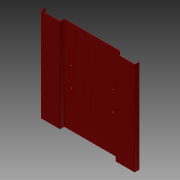
# Autodesk Inventor part: foot
Saved by Autodesk Inventor 2014 SP2 (Build 180246200, 246)
## iProperties
Created: 2016-09-27
Part Number: foot
Material: Steel, Mild
Document SubType Name: Sheet Metal
Designer: cruiser
Density: 7.86 g/cm^3
Sheet Metal Rule: Default_mm
Appearance: Red
Mass: 553.617 g
Surface Area: 901.353 cm^2
Volume: 70.4348 cm^3
Flat Pattern Width: 19.6 cm
Flat Pattern Length: 23.0315 cm
Flat Pattern Area: 451.417 cm^2
Sheet Metal Width: 196.000 mm
Sheet Metal Length: 230.315 mm
Sheet Metal Area: 45141.652 mm^2
Author: cruiser
Autodesk Inventor part; units mm, degrees
ref_plane "YZ Plane" through (0, 0, 0) normal (1, 0, 0) x (0, 1, 0)
ref_plane "XZ Plane" through (0, 0, 0) normal (0, 1, 0) x (-1, 0, 0)
ref_plane "XY Plane" through (0, 0, 0) normal (0, 0, 1) x (1, 0, 0)
sketch "Sketch1" plane through (0, 0, 0) normal (0, 1, 0) x (-1, 0, 0)
  line L0 (-59, -98) -> (59, -98)
  line L1 (59, -98) -> (59, 98)
  line L2 (59, 98) -> (-59, 98)
  line L3 (-59, 98) -> (-59, -98)
  line L4 (-59, -98) -> (59, 98) construction
  line L5 (59, -98) -> (-59, 98) construction
  point P0 (0, 0)
  dimension "d0" = 118
  dimension "d1" = 196
  measures "d0" distance of L2.end L1.end
  measures "d1" distance of L1.end L0.end
extrude "Plate1" add sketch "Sketch1" along normal blind 0.9119
sketch "Sketch2" plane through (58.0881, 0.9119, 98) normal (1, 0, 0) x (0, 1, 0)
  line L0 (0, -196) -> (0, 0)
  line L1 (0, 0) -> (-10, 0)
  line L2 (-10, 0) -> (-10, -196)
  line L3 (-10, -196) -> (0, -196)
  constraints: 6 end point, 1 horizontal, 1 perpendicular, 1 vertical
edge flange "Flange1" height 10 angle 90 thickness 0.9119 bend radius 0.9119 thickness toward (1, 0, 0) relief tear relief width 0.9119 relief depth 0.4559 corner gap 0.9119 corner form 0 edges at (59, 0, 0) (-59, 0, 0) wall of the first edge with corners at (58.0881, 0.9119, -98) (58.0881, 0.9119, 98) (58.0881, -9.0881, 98) (58.0881, -9.0881, -98)
bend "Bend1"
corner "Corner1"
sketch "Sketch3" plane through (58.0881, -8.1763, -98) normal (0, -1, 0) x (1, 0, 0)
  line L0 (0, 196) -> (0, 0)
  line L1 (0, 0) -> (40, 0)
  line L2 (40, 0) -> (40, 196)
  line L3 (40, 196) -> (0, 196)
  constraints: 6 end point, 1 horizontal, 1 perpendicular, 1 vertical
edge flange "Flange2" height 40 angle 90 thickness 0.9119 bend radius 0.9119 thickness toward (0, -1, 0) relief tear relief width 0.9119 relief depth 0.4559 corner gap 0.9119 corner form 0 edges at (59, -9.0881, 0) (-59, -9.0881, 0) wall of the first edge with corners at (58.0881, -8.1763, 98) (58.0881, -8.1763, -98) (98.0881, -8.1763, -98) (98.0881, -8.1763, 98)
bend "Bend2"
corner "Corner2"
sketch "Sketch4" plane through (98.0881, -8.1763, -98) normal (1, 0, 0) x (0, 1, 0)
  line L0 (0, 196) -> (0, 0)
  line L1 (0, 0) -> (9.0881, 0)
  line L2 (9.0881, 0) -> (9.0881, 196)
  line L3 (9.0881, 196) -> (0, 196)
  constraints: 6 end point, 1 horizontal, 1 perpendicular, 1 vertical
edge flange "Flange3" height 10 angle 90 thickness 0.9119 bend radius 0.9119 thickness toward (1, 0, 0) relief tear relief width 0.9119 relief depth 0.4559 corner gap 0.9119 corner form 0 edges at (98.0881, -8.1763, 0) (-98.0881, -8.1763, 0) wall of the first edge with corners at (98.0881, -8.1763, 98) (98.0881, -8.1763, -98) (98.0881, 0.9119, -98) (98.0881, 0.9119, 98)
bend "Bend3"
corner "Corner3"
sketch "Sketch5" plane through (0, 0.9119, 0) normal (0, 1, 0) x (1, 0, 0)
  line L0 (0, 0) -> (-59, 0)
  line L1 (-59, 0) -> (-59, 98)
  line L2 (-59, 98) -> (0, 98)
  line L3 (0, 98) -> (0, 0)
  line L4 (140, -28) -> (-140, -28)
  line L5 (-140, -28) -> (-140, 28)
  line L6 (-140, 28) -> (140, 28)
  line L7 (140, 28) -> (140, -28)
  line L8 (140, -28) -> (-140, 28) construction
  line L9 (-140, -28) -> (140, 28) construction
  circle A0 centre (-44, 20.5) radius 1.5
  circle A1 centre (44, 20.5) radius 1.5
  circle A2 centre (-44, -20.5) radius 1.5
  circle A3 centre (44, -20.5) radius 1.5
  dimension "d34" = 280
  dimension "d35" = 56
  dimension "d36" = 3
  dimension "d38" = 44
  dimension "d41" = 20.5
  constraints: 20 end point, 4 centre point, 4 parallel, 3 symmetric about line, 2 horizontal, 2 midpoint, 2 perpendicular, 3 other
  measures "d34" distance of L5.end L6.end
  measures "d35" distance of L4.end L5.end
  measures "d36" diameter of A0
  measures "d38" distance from line of L3 A0.centre
  measures "d41" distance from line of L0 A0.centre
extrude "Cut1" cut sketch "Sketch5" against normal blind 0.9119 contours A0 | A1 | A2 | A3
fillet "Corner Round1" radius 1 4 edges at (-98.5441, 0.9119, 98) (-98.5441, 0.9119, -98) (98.5441, 0.9119, -98) (98.5441, 0.9119, 98)
equation "\"d0\" = foot_x - 2 * frame_border"
equation "\"d1\" = foot_y"
equation "\"d34\" = frame_front_x"
equation "\"d35\" = frame_front_y"
equation "\"d36\" = m3_diameter"
equation "\"d38\" = laser_offset_x - frame_front_fold"
equation "\"d41\" = 0.5 * frame_front_y - 0.5 * frame_front_fold"
equation "\"d39\" = Thickness"
equation "\"d33\" = corner_small_r"
equation "\"Thickness\" = foot_t"
equation "\"d3\" = BendReliefWidth"
equation "\"d4\" = BendReliefDepth"
equation "\"d5\" = MinimumRemnant"
equation "\"d6\" = BendRadius"
equation "\"d7\" = foot_z"
equation "\"d9\" = BendRadius"
equation "\"d10\" = CornerReliefSize"
equation "\"d11\" = GapSize"
equation "\"d12\" = JacobiRadiusSize"
equation "\"d13\" = BendReliefWidth"
equation "\"d14\" = BendReliefDepth"
equation "\"d15\" = MinimumRemnant"
equation "\"d16\" = BendRadius"
equation "\"d17\" = frame_border"
equation "\"d19\" = BendRadius"
equation "\"d20\" = CornerReliefSize"
equation "\"d21\" = GapSize"
equation "\"d22\" = JacobiRadiusSize"
equation "\"d23\" = BendReliefWidth"
equation "\"d24\" = BendReliefDepth"
equation "\"d25\" = MinimumRemnant"
equation "\"d26\" = BendRadius"
equation "\"d27\" = foot_z"
equation "\"d29\" = BendRadius"
equation "\"d30\" = CornerReliefSize"
equation "\"d31\" = GapSize"
equation "\"d32\" = JacobiRadiusSize"
equation "\"BendRadius\" = Thickness"
equation "\"BendReliefWidth\" = Thickness"
equation "\"BendReliefDepth\" = 0.5 * Thickness"
equation "\"CornerReliefSize\" = 4 * Thickness"
equation "\"MinimumRemnant\" = 2 * Thickness"
equation "\"TransitionRadius\" = BendRadius"
equation "\"JacobiRadiusSize\" = BendRadius"
equation "\"GapSize\" = Thickness"
equation "\"laserresin\" = 5"
equation "\"st1_thickness\" = 0.91186"
equation "\"st2_thickness\" = 1.5875"
equation "\"al1_thickness\" = 0.79375"
equation "\"al2_thickness\" = 1.5875"
equation "\"bend_factor\" = 2.26205"
equation "\"st1_bend\" = 2.06267"
equation "\"st2_bend\" = 3.591"
equation "\"st3_bend\" = 113.10236"
equation "\"al1_bend\" = 1.7955"
equation "\"al2_bend\" = 3.591"
equation "\"al3_bend\" = 113.10236"
equation "\"acrylic1_thickness\" = 5.88"
equation "\"acrylic2_thickness\" = 3.15"
equation "\"acrylic3_thickness\" = 3.15"
equation "\"corner_small_r\" = 1"
equation "\"corner_big_r\" = 5"
equation "\"linear_bearing_spacing\" = 208"
equation "\"galvo_y_out_offset\" = 27"
equation "\"galvo_y_in_offset\" = 17.5"
equation "\"laser_diameter\" = 13"
equation "\"nema17_x\" = 43"
equation "\"nema17_shaft\" = 24"
equation "\"lmk8uu_x\" = 25"
equation "\"lmk8uu_shaft\" = 15"
equation "\"lmk8uu_z\" = 24"
equation "\"shf8_y\" = 43"
equation "\"acme_nut_d\" = 19.1"
equation "\"acme_nut_upper_d\" = 12.7"
equation "\"handle_spacing\" = 50.8"
equation "\"handle_d\" = 4.7625"
equation "\"handle_hole_d\" = 2.845"
equation "\"handle_projection\" = 20.6375"
equation "\"switch_spacing\" = 19"
equation "\"laser_body_diameter\" = 12"
equation "\"m3_diameter\" = 3"
equation "\"m3_head\" = 6"
equation "\"m4_diameter\" = 4"
equation "\"m5_diameter\" = 5"
equation "\"m5_head\" = 10.3"
equation "\"rivet1_diameter\" = 3.26"
equation "\"rivet2_diameter\" = 3.26"
equation "\"brass_insert_drill\" = 4"
equation "\"m5_brass_insert_drill\" = 6.7"
equation "\"m3_press_nut_drill\" = 4.24"
equation "\"m5_press_nut_drill\" = 6.35"
equation "\"platform_t\" = 1.5875"
equation "\"platform_z\" = 65"
equation "\"platform_fold_x\" = 15"
equation "\"platform_crane_gap\" = 0.1"
equation "\"platform_gap\" = 0.1"
equation "\"platform_upper_y\" = 46.625"
equation "\"crane_t\" = 1.5875"
equation "\"crane_x\" = 233"
equation "\"crane_gap\" = 0.1"
equation "\"tray_t\" = 5.88"
equation "\"tray_to_platform_oversize\" = 0"
equation "\"reservoir_t\" = 0.91186"
equation "\"reservoir_z\" = 35"
equation "\"reservoir_flap_y\" = 20.91186"
equation "\"frame_front_t\" = 0.91186"
equation "\"frame_front_x\" = 280"
equation "\"frame_front_y\" = 56"
equation "\"frame_front_fold\" = 15"
equation "\"frame_gap\" = 0.1"
equation "\"frame_back_t\" = 0.91186"
equation "\"frame_back_x\" = 277.97628"
equation "\"frame_back_y\" = 53.97628"
equation "\"frame_back_z\" = 497.97628"
equation "\"drawer_t\" = 0.91186"
equation "\"drawer_gap\" = 0.1"
equation "\"drawer_reservoir_overlap_x\" = 24.08814"
equation "\"drawer_x\" = 202.02372"
equation "\"drawer_y\" = 73"
equation "\"drawer_seal_y\" = 101"
equation "\"drawer_window_gap\" = 6"
equation "\"foot_t\" = 0.91186"
equation "\"foot_x\" = 198"
equation "\"foot_y\" = 196"
equation "\"laser_holder_t\" = 0.91186"
equation "\"laser_holder_z\" = 75"
equation "\"laser_offset_x\" = 59"
equation "\"laser_offset_y\" = 8.5"
equation "\"subframe_t\" = 0.79375"
equation "\"subframe_x\" = 66"
equation "\"subframe_y\" = 55"
equation "\"d2\" = BendRadius"
equation "\"shield_y\" = 71"
equation "\"shield_x\" = 200.2"
equation "\"shield_z\" = 259.9"
equation "\"shield_t\" = 3.15"
equation "\"magnet_t\" = 1.6"
equation "\"magnet_w\" = 12.8"
equation "\"sae_4_40_diameter\" = 2.845"
equation "\"frame_border\" = 40"
equation "\"foot_z\" = 10"
body "Solid1"
